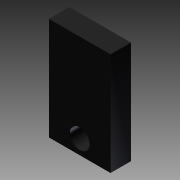
# Autodesk Inventor part: QTR1A
Saved by Autodesk Inventor 2012 (Build 160160000, 160)
## iProperties
Created: 2012-03-28
Part Number: QTR1A
Material: Default
Document SubType Name: Modeling
Designer: Admin
Density: 1 g/cm^3
Mass: 0.233945 g
Surface Area: 3.06892 cm^2
Volume: 0.233945 cm^3
Author: Admin
Autodesk Inventor part; units mm, degrees
ref_plane "YZ Plane" through (0, 0, 0) normal (1, 0, 0) x (0, 1, 0)
ref_plane "XZ Plane" through (0, 0, 0) normal (0, 1, 0) x (-1, 0, 0)
ref_plane "XY Plane" through (0, 0, 0) normal (0, 0, 1) x (1, 0, 0)
sketch "Sketch1" plane through (0, 0, 0) normal (0, 0, 1) x (1, 0, 0)
  line L0 (0, 0) -> (7.62, 0)
  line L1 (7.62, 0) -> (7.62, -12.7)
  line L2 (7.62, -12.7) -> (0, -12.7)
  line L3 (0, -12.7) -> (0, 0)
  dimension "d0" = 7.62
  dimension "d1" = 12.7
  constraints: 8 end point, 2 parallel, 1 horizontal, 1 perpendicular
  measures "d0" distance of L1.end L2.end
  measures "d1" distance of L0.end L1.end
extrude "Extrusion1" add sketch "Sketch1" along normal blind 2.54
sketch "Sketch2" plane through (0, 0, 2.54) normal (0, 0, 1) x (1, 0, 0)
  line L0 (7.62, 0) -> (7.62, -12.7) projected
  line L1 (7.62, -12.7) -> (0, -12.7) projected
  point P0 (3.81, -10.922)
  dimension "d4" = 3.81
  dimension "d5" = 1.778
  measures "d4" distance from line of L0 point (3.81, -10.922)
  measures "d5" distance from line of L1 point (3.81, -10.922)
hole "Hole1" at (3.81, -10.922, 2.54) direction (0, 0, -1) diameter 2.4384 depth 5.2203 tip angle 118 clearance for "Flat Head Machine Screw (82)" size "#2" standard "Ansi Unified Screw Threads"
sketch "Sketch3" plane through (0, -12.7, 0) normal (0, -1, 0) x (1, 0, 0)
  point P0 (2.8575, -69.85)
  point P1 (2.8575, -44.45)
  point P2 (2.8575, -19.304)
  point P3 (-70.8025, -30.48)
  point P4 (-70.8025, -10.16)
  point P5 (-109.5375, -30.48)
  point P6 (-109.5375, -10.16)
  point P7 (-183.1975, -19.304)
  point P8 (-183.1975, -44.45)
  point P9 (-183.1975, -69.85)
body "Solid1"
